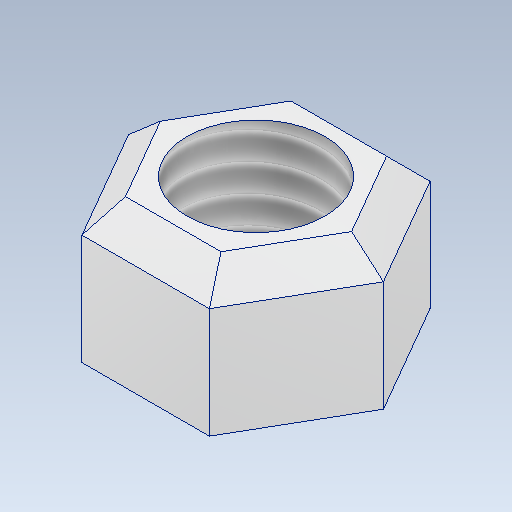
# Autodesk Inventor part: M5_nut_5mm
Saved by Autodesk Inventor 2020.3 (Build 243373000, 373)
## iProperties
Created: 2021-03-23
Part Number: M5_nut_5mm
Material: Aluminium 6061
Document SubType Name: Modeling
Designer: patry
Density: 2.7 g/cm^3
Appearance: Aluminium — płaski
Mass: 0.448879 g
Surface Area: 2.71017 cm^2
Volume: 0.166252 cm^3
Author: patry
Autodesk Inventor part; units mm, degrees
ref_plane "YZ Plane" through (0, 0, 0) normal (1, 0, 0) x (0, 1, 0)
ref_plane "XZ Plane" through (0, 0, 0) normal (0, 1, 0) x (-1, 0, 0)
ref_plane "XY Plane" through (0, 0, 0) normal (0, 0, 1) x (1, 0, 0)
sketch "Szkic1" plane through (0, 0, 0) normal (0, 1, 0) x (-1, 0, 0)
  line L0 (-2.3094, -4) -> (-4.6188, 0)
  line L1 (-4.6188, 0) -> (-2.3094, 4)
  line L2 (-2.3094, 4) -> (2.3094, 4)
  line L3 (2.3094, 4) -> (4.6188, 0)
  line L4 (4.6188, 0) -> (2.3094, -4)
  line L5 (2.3094, -4) -> (-2.3094, -4)
  circle A0 centre (0, 0) radius 2.5
  dimension "d0" = 8
  dimension "d1" = 5
  constraints: 12 end point, 2 coincident, 1 centre point, 13 other
  measures "d0" distance between parallel lines of L2 L5
  measures "d1" diameter of A0
extrude "Wyciągnięcie proste1" add sketch "Szkic1" along normal blind 5
thread "Gwint1" size "M6x1" class "6H" standard "ANSI Metric M Profile" length 5
chamfer "Faza1" distance 1 angle 45 6 edges at (-3.4641, 5, 2) (0, 5, 4) (3.4641, 5, 2) (3.4641, 5, -2) (0, 5, -4) (-3.4641, 5, -2)
